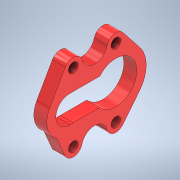
# Autodesk Inventor part: hw9
Saved by Autodesk Inventor 2021 (Build 250183000, 183)
## iProperties
Created: 2022-04-30
Part Number: hw9
Material: Generic
Document SubType Name: Modeling
Designer: authe
Density: 1 g/cm^3
Appearance: Light Red
Author: authe
Autodesk Inventor part; units mm, degrees
ref_plane "YZ Plane" through (0, 0, 0) normal (1, 0, 0) x (0, 1, 0)
ref_plane "XZ Plane" through (0, 0, 0) normal (0, 1, 0) x (-1, 0, 0)
ref_plane "XY Plane" through (0, 0, 0) normal (0, 0, 1) x (1, 0, 0)
sketch "Sketch1" plane through (0, 0, 0) normal (1, 0, 0) x (0, 1, 0)
  arc A0 (17.2522, 102.4526) -> (0, 107) centre (0, 72) ccw
  arc A1 (0, -47) -> (29.2642, -36.7778) centre (0, 0) ccw
  arc A2 (56.3935, 52.3189) -> (59.948, 78.2643) centre (53, 66) ccw
  arc A3 (61.6337, -11.0214) -> (56.3309, 13.511) centre (52.9167, -0.0663) ccw
  line L0 (17.2522, 102.4526) -> (59.948, 78.2643)
  line L1 (61.6337, -11.0214) -> (29.2642, -36.7778)
  arc A4 (56.3935, 52.3189) -> (56.3309, 13.511) centre (61.2084, 32.9071) ccw
  arc A5 (21, 72) -> (0, 93) centre (0, 72) ccw
  arc A6 (0, -32.5) -> (21, 24.8042) centre (0, 0) ccw
  line L2 (21, 72) -> (21, 30.8042)
  circle A7 centre (53, 66) radius 7.5
  circle A8 centre (52.9167, -0.0663) radius 7.5
  arc A9 (-56.3704, 13.5882) -> (-56.3704, 52.4118) centre (-61.1854, 33) ccw
  line L3 (-20.9781, 66) -> (-21, 24.8042)
  circle A10 centre (-53, 66) radius 7.5
  line L4 (-28.9912, 91.6089) -> (-58.5472, 78.8541)
  arc A11 (0, 107) -> (-28.9912, 91.6089) centre (0, 72) ccw
  arc A12 (-58.5472, 78.8541) -> (-56.3704, 52.4118) centre (-53, 66) ccw
  arc A13 (-56.3704, 13.5882) -> (-61.717, -10.9551) centre (-53, 0) ccw
  arc A14 (-21, 24.8042) -> (0, -32.5) centre (0, 0) ccw
  arc A15 (-29.2642, -36.7778) -> (0, -47) centre (0, 0) ccw
  line L5 (-61.717, -10.9551) -> (-29.2642, -36.7778)
  circle A16 centre (-53, 0) radius 7.5
  arc A17 (0, 93) -> (-20.9781, 71.0401) centre (0, 72) ccw
  line L6 (21, 30.8042) -> (21, 24.8042)
  line L7 (-20.9781, 71.0401) -> (-20.9781, 66)
  dimension "d15" = 15
  dimension "d16" = 20
  dimension "d17" = 32.5
  dimension "d18" = 47
  dimension "d19" = 21
  dimension "d20" = 72
  dimension "d21" = 106
  dimension "d22" = 66
  dimension "d23" = 15
  constraints: 28 point on circle, 18 centre point, 16 end point, 9 coincident, 7 tangent, 2 vertical, 1 parallel
  measures "d15" diameter of A8
  measures "d16" radius of A4
  measures "d17" radius of A6
  measures "d18" radius of A15
  measures "d19" radius of A5
  measures "d20" distance of A15.centre A11.centre
  measures "d21" distance of A12.centre A2.centre
  measures "d22" distance of A16.centre A12.centre
  measures "d23" diameter of A7
extrude "Extrusion1" add sketch "Sketch1" against normal mid plane 20
body "Solid1"
